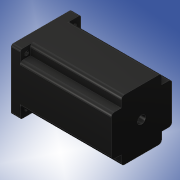
# Autodesk Inventor part: Part1
Saved by Autodesk Inventor 2017 SP1 (Build 210196100, 196)
## iProperties
Created: 2017-08-05
Part Number: Part1
Material: Steel, Carbon
Document SubType Name: Modeling
Designer: Zach
Density: 7.85 g/cm^3
Appearance: Glossy - Black
Author: Zach
Autodesk Inventor part; units mm, degrees
ref_plane "YZ Plane" through (0, 0, 0) normal (1, 0, 0) x (0, 1, 0)
ref_plane "XZ Plane" through (0, 0, 0) normal (0, 1, 0) x (-1, 0, 0)
ref_plane "XY Plane" through (0, 0, 0) normal (0, 0, 1) x (1, 0, 0)
sketch "Sketch2" plane through (0, 0, 0) normal (0, 0, 1) x (1, 0, 0)
  line L0 (0, 0) -> (99, 0)
  line L1 (99, 0) -> (99, 60)
  line L2 (99, 60) -> (0, 60)
  line L3 (0, 60) -> (0, 0)
  dimension "d2" = 99
  dimension "d3" = 60
  constraints: 8 end point, 2 parallel, 1 horizontal, 1 perpendicular
  measures "d2" distance of L2.end L1.end
  measures "d3" distance of L1.end L0.end
extrude "Extrusion1" add sketch "Sketch2" along normal blind 60
sketch "Sketch3" plane through (0, 0, 0) normal (-1, 0, 0) x (0, 0, 1)
  circle A0 centre (30, 30) radius 4
  line L0 (0, 60) -> (60, 60) projected
  line L1 (0, 60) -> (0, 0) projected
  point P0 (30, 60)
  point P1 (0, 30)
  dimension "d6" = 8
  constraints: 2 midpoint, 1 centre point, 1 horizontal alignment, 1 vertical alignment
  measures "d6" diameter of A0
extrude "Extrusion2" cut sketch "Sketch3" against normal through all
sketch "Sketch4" plane through (99, 0, 0) normal (1, 0, 0) x (0, 0, -1)
  line L0 (0, 60) -> (-60, 60) projected
  line L1 (-60, 60) -> (-50, 60)
  line L2 (-50, 60) -> (-50, 50)
  line L3 (-50, 50) -> (-60, 50)
  line L4 (-60, 50) -> (-60, 60)
  line L5 (0, 60) -> (-10, 60)
  line L6 (-10, 60) -> (-10, 50)
  line L7 (-10, 50) -> (0, 50)
  line L8 (0, 50) -> (0, 60)
  line L9 (0, 0) -> (-10, 0)
  line L10 (-10, 0) -> (-10, 10)
  line L11 (-10, 10) -> (0, 10)
  line L12 (0, 10) -> (0, 0)
  line L13 (-60, 0) -> (-50, 0)
  line L14 (-50, 0) -> (-50, 10)
  line L15 (-50, 10) -> (-60, 10)
  line L16 (-60, 10) -> (-60, 0)
  dimension "d9" = 10
  dimension "d10" = 10
  dimension "d11" = 10
  dimension "d12" = 10
  dimension "d13" = 10
  dimension "d14" = 10
  dimension "d15" = 10
  dimension "d16" = 10
  constraints: 32 end point, 8 parallel, 4 horizontal, 4 perpendicular
  measures "d9" distance of L2.end L3.end
  measures "d10" distance of L1.end L2.end
  measures "d11" distance of L7.end L6.end
  measures "d12" distance of L6.end L5.end
  measures "d13" distance of L10.end L11.end
  measures "d14" distance of L9.end L10.end
  measures "d15" distance of L15.end L14.end
  measures "d16" distance of L14.end L13.end
extrude "Extrusion3" cut sketch "Sketch4" against normal blind 90
fillet "Fillet1" radius 3 8 edges at (54, 50, 60) (54, 60, 50) (54, 60, 10) (54, 50, 0) (54, 10, 60) (54, 0, 50) (54, 0, 10) (54, 10, 0)
fillet "Fillet2" radius 2 4 edges at (4.5, 60, 60) (4.5, 0, 60) (4.5, 60, 0) (4.5, 0, 0)
sketch "Sketch5" plane through (0, 2, 0) normal (-1, 0, 0) x (0, 0, 1)
  circle A0 centre (30, 28) radius 4 projected
  circle A1 centre (30, 28) radius 17.5
  point P0 (0, -2)
  dimension "d21" = 35
  constraints: 1 centre point, 1 coincident
  measures "d21" diameter of A1
extrude "Extrusion4" add sketch "Sketch5" along normal blind 3
sketch "Sketch6" plane through (0, 2, 0) normal (-1, 0, 0) x (0, 0, 1)
  line L0 (6.4, 4.4) -> (53.6, 4.4) construction
  line L1 (53.6, 4.4) -> (53.6, 51.6) construction
  line L2 (53.6, 51.6) -> (6.4, 51.6) construction
  line L3 (6.4, 51.6) -> (6.4, 4.4) construction
  circle A0 centre (6.4, 51.6) radius 2
  circle A1 centre (53.6, 51.6) radius 2
  circle A2 centre (53.6, 4.4) radius 2
  circle A3 centre (6.4, 4.4) radius 2
  circle A4 centre (30, 28) radius 4 construction
  point P0 (0, -2)
  point P1 (30, 51.6)
  point P2 (53.6, 28)
  dimension "d24" = 47.2
  dimension "d25" = 47.2
  dimension "d26" = 4
  dimension "d27" = 4
  dimension "d28" = 4
  dimension "d29" = 4
  constraints: 8 end point, 4 centre point, 4 coincident, 2 midpoint, 2 parallel, 1 horizontal, 1 horizontal alignment, 1 perpendicular, 1 vertical alignment
  measures "d24" distance of L2.end L1.end
  measures "d25" distance of L1.end L0.end
  measures "d26" diameter of A0
  measures "d27" diameter of A1
  measures "d28" diameter of A2
  measures "d29" diameter of A3
extrude "Extrusion5" cut sketch "Sketch6" against normal through all
body "Solid1"
